Autodesk Fusion 360 part; units mm, degrees
(part 11 of 18)
sketch "Sketch1 (2)" plane through (0, 0, 0) normal (0, 0, 1) x (1, 0, 0) in component "Component"
  spline S0 degree 5 poles (24.241, -1.3145) (24.2412, -1.3145) (24.2415, -1.3145) (24.242, -1.3146) (24.2429, -1.3146) (24.2442, -1.3146) (24.2456, -1.3147) (24.2473, -1.3147) (24.2491, -1.3148) (24.2512, -1.3148) (24.2534, -1.3149) (24.2558, -1.3149) (24.2584, -1.315) (24.2611, -1.315) (24.2641, -1.3151) (24.2672, -1.3151) (24.2704, -1.3151) (24.2739, -1.3151) (24.2775, -1.3151) (24.2812, -1.3151) (24.2851, -1.3151) (24.2892, -1.315) (24.2934, -1.315) (24.2977, -1.3149) (24.3022, -1.3149) (24.3069, -1.3148) (24.3117, -1.3147) (24.3166, -1.3145) (24.3216, -1.3144) (24.3268, -1.3143) (24.3322, -1.3141) (24.3376, -1.3139) (24.3432, -1.3137) (24.3489, -1.3135) (24.3548, -1.3132) (24.3608, -1.313) (24.3669, -1.3127) (24.3731, -1.3124) (24.3794, -1.312) (24.3859, -1.3117) (24.3924, -1.3113) (24.3991, -1.3109) (24.4059, -1.3105) (24.4129, -1.3101) (24.4199, -1.3096) (24.427, -1.3091) (24.4343, -1.3086) (24.4416, -1.308) (24.4491, -1.3075) (24.4567, -1.3069) (24.4644, -1.3062) (24.4721, -1.3056) (24.48, -1.3049) (24.488, -1.3042) (24.4961, -1.3035) (24.5043, -1.3027) (24.5126, -1.3019) (24.521, -1.3011) (24.5294, -1.3003) (24.538, -1.2994) (24.5467, -1.2985) (24.5554, -1.2976) (24.5643, -1.2966) (24.5732, -1.2956) (24.5823, -1.2946) (24.5914, -1.2935) (24.6006, -1.2925) (24.6099, -1.2913) (24.6193, -1.2902) (24.6288, -1.289) (24.6383, -1.2878) (24.648, -1.2865) (24.6577, -1.2853) (24.6675, -1.284) (24.6774, -1.2826) (24.6874, -1.2812) (24.6974, -1.2798) (24.7076, -1.2784) (24.7178, -1.2769) (24.7281, -1.2754) (24.7385, -1.2738) (24.7489, -1.2723) (24.7594, -1.2707) (24.77, -1.269) (24.7807, -1.2673) (24.7915, -1.2656) (24.8023, -1.2638) (24.8132, -1.2621) (24.8242, -1.2602) (24.8352, -1.2584) (24.8464, -1.2565) (24.8575, -1.2545) (24.8688, -1.2526) (24.8801, -1.2506) (24.8915, -1.2485) (24.903, -1.2464) (24.9146, -1.2443) (24.9262, -1.2422) (24.9378, -1.24) (24.9496, -1.2378) (24.9614, -1.2355) (24.9733, -1.2332) (24.9852, -1.2308) (24.9972, -1.2285) (25.0093, -1.226) (25.0214, -1.2236) (25.0336, -1.2211) (25.0458, -1.2186) (25.0581, -1.216) (25.0705, -1.2134) (25.083, -1.2107) (25.0955, -1.2081) (25.108, -1.2053) (25.1206, -1.2026) (25.1333, -1.1998) (25.1461, -1.1969) (25.1589, -1.194) (25.1717, -1.1911) (25.1846, -1.1882) (25.1976, -1.1852) (25.2106, -1.1821) (25.2237, -1.179) (25.2368, -1.1759) (25.25, -1.1728) (25.2633, -1.1696) (25.2766, -1.1663) (25.2899, -1.163) (25.3034, -1.1597) (25.3168, -1.1564) (25.3303, -1.153) (25.3439, -1.1495) (25.3575, -1.146) (25.3712, -1.1425) (25.3849, -1.1389) (25.3987, -1.1353) (25.4125, -1.1317) (25.4264, -1.128) (25.4403, -1.1243) (25.4543, -1.1205) (25.4683, -1.1167) (25.4824, -1.1128) (25.4965, -1.1089) (25.5107, -1.105) (25.5249, -1.101) (25.5392, -1.097) (25.5535, -1.0929) (25.5679, -1.0888) (25.5823, -1.0846) (25.5967, -1.0805) (25.6112, -1.0762) (25.6258, -1.0719) (25.6404, -1.0676) (25.655, -1.0633) (25.6697, -1.0589) (25.6844, -1.0544) (25.6992, -1.0499) (25.714, -1.0454) (25.7288, -1.0408) (25.7437, -1.0362) (25.7587, -1.0316) (25.7736, -1.0268) (25.7887, -1.0221) (25.8037, -1.0173) (25.8188, -1.0125) (25.834, -1.0076) (25.8492, -1.0027) (25.8644, -0.9977) (25.8797, -0.9927) (25.895, -0.9877) (25.9103, -0.9826) (25.9257, -0.9775) (25.9411, -0.9723) (25.9566, -0.9671) (25.9721, -0.9618) (25.9876, -0.9565) (26.0032, -0.9511) (26.0188, -0.9457) (26.0345, -0.9403) (26.0502, -0.9348) (26.0659, -0.9293) (26.0817, -0.9237) (26.0975, -0.9181) (26.1133, -0.9124) (26.1292, -0.9067) (26.1451, -0.901) (26.161, -0.8952) (26.177, -0.8894) (26.193, -0.8835) (26.2091, -0.8776) (26.2252, -0.8716) (26.2413, -0.8656) (26.2574, -0.8595) (26.2736, -0.8534) (26.2898, -0.8473) (26.3061, -0.8411) (26.3224, -0.8349) (26.3387, -0.8286) (26.355, -0.8223) (26.3714, -0.8159) (26.3878, -0.8095) (26.4043, -0.803) (26.4207, -0.7965) (26.4373, -0.79) (26.4538, -0.7834) (26.4704, -0.7768) (26.487, -0.7701) (26.5036, -0.7633) (26.5202, -0.7566) (26.5369, -0.7498) (26.5537, -0.7429) (26.5704, -0.736) (26.5872, -0.7291) (26.604, -0.7221) (26.6208, -0.715) (26.6377, -0.7079) (26.6546, -0.7008) (26.6715, -0.6936) (26.6884, -0.6864) (26.7054, -0.6792) (26.7224, -0.6718) (26.7394, -0.6645) (26.7565, -0.6571) (26.7736, -0.6496) (26.7907, -0.6422) (26.8078, -0.6346) (26.825, -0.627) (26.8422, -0.6194) (26.8594, -0.6117) (26.8766, -0.604) (26.8939, -0.5963) (26.9112, -0.5885) (26.9285, -0.5806) (26.9458, -0.5727) (26.9632, -0.5648) (26.9806, -0.5568) (26.998, -0.5488) (27.0154, -0.5407) (27.0329, -0.5325) (27.0504, -0.5244) (27.0679, -0.5162) (27.0854, -0.5079) (27.0995, -0.5013) (27.11, -0.4963) (27.117, -0.4929) (27.1206, -0.4912) knots 0 0 0 0 0 0 0.00416667 0.00833333 0.0125 0.01666667 0.02083333 0.025 0.02916667 0.03333333 0.0375 0.04166667 0.04583333 0.05 0.05416667 0.05833333 0.0625 0.06666667 0.07083333 0.075 0.07916667 0.08333333 0.0875 0.09166667 0.09583333 0.1 0.10416667 0.10833333 0.1125 0.11666667 0.12083333 0.125 0.12916667 0.13333333 0.1375 0.14166667 0.14583333 0.15 0.15416667 0.15833333 0.1625 0.16666667 0.17083333 0.175 0.17916667 0.18333333 0.1875 0.19166667 0.19583333 0.2 0.20416667 0.20833333 0.2125 0.21666667 0.22083333 0.225 0.22916667 0.23333333 0.2375 0.24166667 0.24583333 0.25 0.25416667 0.25833333 0.2625 0.26666667 0.27083333 0.275 0.27916667 0.28333333 0.2875 0.29166667 0.29583333 0.3 0.30416667 0.30833333 0.3125 0.31666667 0.32083333 0.325 0.32916667 0.33333333 0.3375 0.34166667 0.34583333 0.35 0.35416667 0.35833333 0.3625 0.36666667 0.37083333 0.375 0.37916667 0.38333333 0.3875 0.39166667 0.39583333 0.4 0.40416667 0.40833333 0.4125 0.41666667 0.42083333 0.425 0.42916667 0.43333333 0.4375 0.44166667 0.44583333 0.45 0.45416667 0.45833333 0.4625 0.46666667 0.47083333 0.475 0.47916667 0.48333333 0.4875 0.49166667 0.49583333 0.5 0.50416667 0.50833333 0.5125 0.51666667 0.52083333 0.525 0.52916667 0.53333333 0.5375 0.54166667 0.54583333 0.55 0.55416667 0.55833333 0.5625 0.56666667 0.57083333 0.575 0.57916667 0.58333333 0.5875 0.59166667 0.59583333 0.6 0.60416667 0.60833333 0.6125 0.61666667 0.62083333 0.625 0.62916667 0.63333333 0.6375 0.64166667 0.64583333 0.65 0.65416667 0.65833333 0.6625 0.66666667 0.67083333 0.675 0.67916667 0.68333333 0.6875 0.69166667 0.69583333 0.7 0.70416667 0.70833333 0.7125 0.71666667 0.72083333 0.725 0.72916667 0.73333333 0.7375 0.74166667 0.74583333 0.75 0.75416667 0.75833333 0.7625 0.76666667 0.77083333 0.775 0.77916667 0.78333333 0.7875 0.79166667 0.79583333 0.8 0.80416667 0.80833333 0.8125 0.81666667 0.82083333 0.825 0.82916667 0.83333333 0.8375 0.84166667 0.84583333 0.85 0.85416667 0.85833333 0.8625 0.86666667 0.87083333 0.875 0.87916667 0.88333333 0.8875 0.89166667 0.89583333 0.9 0.90416667 0.90833333 0.9125 0.91666667 0.92083333 0.925 0.92916667 0.93333333 0.9375 0.94166667 0.94583333 0.95 0.95416667 0.95833333 0.9625 0.96666667 0.97083333 0.975 0.97916667 0.98333333 0.9875 0.99166667 0.99583333 1 1 1 1 1 1
  spline S1 degree 5 poles (24.241, 1.3145) (24.2412, 1.3145) (24.2415, 1.3145) (24.242, 1.3146) (24.2429, 1.3146) (24.2442, 1.3146) (24.2456, 1.3147) (24.2473, 1.3147) (24.2491, 1.3148) (24.2512, 1.3148) (24.2534, 1.3149) (24.2558, 1.3149) (24.2584, 1.315) (24.2611, 1.315) (24.2641, 1.3151) (24.2672, 1.3151) (24.2704, 1.3151) (24.2739, 1.3151) (24.2775, 1.3151) (24.2812, 1.3151) (24.2851, 1.3151) (24.2892, 1.315) (24.2934, 1.315) (24.2977, 1.3149) (24.3022, 1.3149) (24.3069, 1.3148) (24.3117, 1.3147) (24.3166, 1.3145) (24.3216, 1.3144) (24.3268, 1.3143) (24.3322, 1.3141) (24.3376, 1.3139) (24.3432, 1.3137) (24.3489, 1.3135) (24.3548, 1.3132) (24.3608, 1.313) (24.3669, 1.3127) (24.3731, 1.3124) (24.3794, 1.312) (24.3859, 1.3117) (24.3924, 1.3113) (24.3991, 1.3109) (24.4059, 1.3105) (24.4129, 1.3101) (24.4199, 1.3096) (24.427, 1.3091) (24.4343, 1.3086) (24.4416, 1.308) (24.4491, 1.3075) (24.4567, 1.3069) (24.4644, 1.3062) (24.4721, 1.3056) (24.48, 1.3049) (24.488, 1.3042) (24.4961, 1.3035) (24.5043, 1.3027) (24.5126, 1.3019) (24.521, 1.3011) (24.5294, 1.3003) (24.538, 1.2994) (24.5467, 1.2985) (24.5554, 1.2976) (24.5643, 1.2966) (24.5732, 1.2956) (24.5823, 1.2946) (24.5914, 1.2935) (24.6006, 1.2925) (24.6099, 1.2913) (24.6193, 1.2902) (24.6288, 1.289) (24.6383, 1.2878) (24.648, 1.2865) (24.6577, 1.2853) (24.6675, 1.284) (24.6774, 1.2826) (24.6874, 1.2812) (24.6974, 1.2798) (24.7076, 1.2784) (24.7178, 1.2769) (24.7281, 1.2754) (24.7385, 1.2738) (24.7489, 1.2723) (24.7594, 1.2707) (24.77, 1.269) (24.7807, 1.2673) (24.7915, 1.2656) (24.8023, 1.2638) (24.8132, 1.2621) (24.8242, 1.2602) (24.8352, 1.2584) (24.8464, 1.2565) (24.8575, 1.2545) (24.8688, 1.2526) (24.8801, 1.2506) (24.8915, 1.2485) (24.903, 1.2464) (24.9146, 1.2443) (24.9262, 1.2422) (24.9378, 1.24) (24.9496, 1.2378) (24.9614, 1.2355) (24.9733, 1.2332) (24.9852, 1.2308) (24.9972, 1.2285) (25.0093, 1.226) (25.0214, 1.2236) (25.0336, 1.2211) (25.0458, 1.2186) (25.0581, 1.216) (25.0705, 1.2134) (25.083, 1.2107) (25.0955, 1.2081) (25.108, 1.2053) (25.1206, 1.2026) (25.1333, 1.1998) (25.1461, 1.1969) (25.1589, 1.194) (25.1717, 1.1911) (25.1846, 1.1882) (25.1976, 1.1852) (25.2106, 1.1821) (25.2237, 1.179) (25.2368, 1.1759) (25.25, 1.1728) (25.2633, 1.1696) (25.2766, 1.1663) (25.2899, 1.163) (25.3034, 1.1597) (25.3168, 1.1564) (25.3303, 1.153) (25.3439, 1.1495) (25.3575, 1.146) (25.3712, 1.1425) (25.3849, 1.1389) (25.3987, 1.1353) (25.4125, 1.1317) (25.4264, 1.128) (25.4403, 1.1243) (25.4543, 1.1205) (25.4683, 1.1167) (25.4824, 1.1128) (25.4965, 1.1089) (25.5107, 1.105) (25.5249, 1.101) (25.5392, 1.097) (25.5535, 1.0929) (25.5679, 1.0888) (25.5823, 1.0846) (25.5967, 1.0805) (25.6112, 1.0762) (25.6258, 1.0719) (25.6404, 1.0676) (25.655, 1.0633) (25.6697, 1.0589) (25.6844, 1.0544) (25.6992, 1.0499) (25.714, 1.0454) (25.7288, 1.0408) (25.7437, 1.0362) (25.7587, 1.0316) (25.7736, 1.0268) (25.7887, 1.0221) (25.8037, 1.0173) (25.8188, 1.0125) (25.834, 1.0076) (25.8492, 1.0027) (25.8644, 0.9977) (25.8797, 0.9927) (25.895, 0.9877) (25.9103, 0.9826) (25.9257, 0.9775) (25.9411, 0.9723) (25.9566, 0.9671) (25.9721, 0.9618) (25.9876, 0.9565) (26.0032, 0.9511) (26.0188, 0.9457) (26.0345, 0.9403) (26.0502, 0.9348) (26.0659, 0.9293) (26.0817, 0.9237) (26.0975, 0.9181) (26.1133, 0.9124) (26.1292, 0.9067) (26.1451, 0.901) (26.161, 0.8952) (26.177, 0.8894) (26.193, 0.8835) (26.2091, 0.8776) (26.2252, 0.8716) (26.2413, 0.8656) (26.2574, 0.8595) (26.2736, 0.8534) (26.2898, 0.8473) (26.3061, 0.8411) (26.3224, 0.8349) (26.3387, 0.8286) (26.355, 0.8223) (26.3714, 0.8159) (26.3878, 0.8095) (26.4043, 0.803) (26.4207, 0.7965) (26.4373, 0.79) (26.4538, 0.7834) (26.4704, 0.7768) (26.487, 0.7701) (26.5036, 0.7633) (26.5202, 0.7566) (26.5369, 0.7498) (26.5537, 0.7429) (26.5704, 0.736) (26.5872, 0.7291) (26.604, 0.7221) (26.6208, 0.715) (26.6377, 0.7079) (26.6546, 0.7008) (26.6715, 0.6936) (26.6884, 0.6864) (26.7054, 0.6792) (26.7224, 0.6718) (26.7394, 0.6645) (26.7565, 0.6571) (26.7736, 0.6496) (26.7907, 0.6422) (26.8078, 0.6346) (26.825, 0.627) (26.8422, 0.6194) (26.8594, 0.6117) (26.8766, 0.604) (26.8939, 0.5963) (26.9112, 0.5885) (26.9285, 0.5806) (26.9458, 0.5727) (26.9632, 0.5648) (26.9806, 0.5568) (26.998, 0.5488) (27.0154, 0.5407) (27.0329, 0.5325) (27.0504, 0.5244) (27.0679, 0.5162) (27.0854, 0.5079) (27.0995, 0.5013) (27.11, 0.4963) (27.117, 0.4929) (27.1206, 0.4912) knots 0 0 0 0 0 0 0.00416667 0.00833333 0.0125 0.01666667 0.02083333 0.025 0.02916667 0.03333333 0.0375 0.04166667 0.04583333 0.05 0.05416667 0.05833333 0.0625 0.06666667 0.07083333 0.075 0.07916667 0.08333333 0.0875 0.09166667 0.09583333 0.1 0.10416667 0.10833333 0.1125 0.11666667 0.12083333 0.125 0.12916667 0.13333333 0.1375 0.14166667 0.14583333 0.15 0.15416667 0.15833333 0.1625 0.16666667 0.17083333 0.175 0.17916667 0.18333333 0.1875 0.19166667 0.19583333 0.2 0.20416667 0.20833333 0.2125 0.21666667 0.22083333 0.225 0.22916667 0.23333333 0.2375 0.24166667 0.24583333 0.25 0.25416667 0.25833333 0.2625 0.26666667 0.27083333 0.275 0.27916667 0.28333333 0.2875 0.29166667 0.29583333 0.3 0.30416667 0.30833333 0.3125 0.31666667 0.32083333 0.325 0.32916667 0.33333333 0.3375 0.34166667 0.34583333 0.35 0.35416667 0.35833333 0.3625 0.36666667 0.37083333 0.375 0.37916667 0.38333333 0.3875 0.39166667 0.39583333 0.4 0.40416667 0.40833333 0.4125 0.41666667 0.42083333 0.425 0.42916667 0.43333333 0.4375 0.44166667 0.44583333 0.45 0.45416667 0.45833333 0.4625 0.46666667 0.47083333 0.475 0.47916667 0.48333333 0.4875 0.49166667 0.49583333 0.5 0.50416667 0.50833333 0.5125 0.51666667 0.52083333 0.525 0.52916667 0.53333333 0.5375 0.54166667 0.54583333 0.55 0.55416667 0.55833333 0.5625 0.56666667 0.57083333 0.575 0.57916667 0.58333333 0.5875 0.59166667 0.59583333 0.6 0.60416667 0.60833333 0.6125 0.61666667 0.62083333 0.625 0.62916667 0.63333333 0.6375 0.64166667 0.64583333 0.65 0.65416667 0.65833333 0.6625 0.66666667 0.67083333 0.675 0.67916667 0.68333333 0.6875 0.69166667 0.69583333 0.7 0.70416667 0.70833333 0.7125 0.71666667 0.72083333 0.725 0.72916667 0.73333333 0.7375 0.74166667 0.74583333 0.75 0.75416667 0.75833333 0.7625 0.76666667 0.77083333 0.775 0.77916667 0.78333333 0.7875 0.79166667 0.79583333 0.8 0.80416667 0.80833333 0.8125 0.81666667 0.82083333 0.825 0.82916667 0.83333333 0.8375 0.84166667 0.84583333 0.85 0.85416667 0.85833333 0.8625 0.86666667 0.87083333 0.875 0.87916667 0.88333333 0.8875 0.89166667 0.89583333 0.9 0.90416667 0.90833333 0.9125 0.91666667 0.92083333 0.925 0.92916667 0.93333333 0.9375 0.94166667 0.94583333 0.95 0.95416667 0.95833333 0.9625 0.96666667 0.97083333 0.975 0.97916667 0.98333333 0.9875 0.99166667 0.99583333 1 1 1 1 1 1
  spline S2 degree 5 poles (24.2398, -1.3145) (24.2398, -1.3145) (24.2399, -1.3145) (24.2401, -1.3145) (24.2403, -1.3145) (24.2405, -1.3145) (24.2407, -1.3145) (24.2409, -1.3145) (24.241, -1.3145) (24.241, -1.3145) knots 0 0 0 0 0 0 0.2 0.4 0.6 0.8 1 1 1 1 1 1
  spline S3 degree 5 poles (24.2398, 1.3145) (24.2398, 1.3145) (24.2399, 1.3145) (24.2401, 1.3145) (24.2403, 1.3145) (24.2405, 1.3145) (24.2407, 1.3145) (24.2409, 1.3145) (24.241, 1.3145) (24.241, 1.3145) knots 0 0 0 0 0 0 0.2 0.4 0.6 0.8 1 1 1 1 1 1
  line L0 (0, 0) -> (24.2398, -1.3145)
  line L1 (0, 0) -> (24.2398, 1.3145)
  arc A0 (27.1206, -0.4912) -> (27.1206, 0.4912) centre (0, 0) ccw
  point P0 (24.2448, -1.3147)
  point P1 (24.2511, -1.3148)
  point P2 (24.2599, -1.315)
  point P3 (24.2712, -1.3151)
  point P4 (24.285, -1.3151)
  point P5 (24.3013, -1.3149)
  point P6 (24.3202, -1.3145)
  point P7 (24.3415, -1.3138)
  point P8 (24.3654, -1.3127)
  point P9 (24.3917, -1.3114)
  point P10 (24.4206, -1.3095)
  point P11 (24.4519, -1.3072)
  point P12 (24.4857, -1.3044)
  point P13 (24.522, -1.301)
  point P14 (24.5607, -1.297)
  point P15 (24.6019, -1.2923)
  point P16 (24.6456, -1.2869)
  point P17 (24.6916, -1.2806)
  point P18 (24.7401, -1.2736)
  point P19 (24.791, -1.2657)
  point P20 (24.8443, -1.2568)
  point P21 (24.9, -1.247)
  point P22 (24.9581, -1.2361)
  point P23 (25.0185, -1.2242)
  point P24 (25.0812, -1.2111)
  point P25 (25.1463, -1.1969)
  point P26 (25.2136, -1.1814)
  point P27 (25.2832, -1.1647)
  point P28 (25.3552, -1.1466)
  point P29 (25.4293, -1.1272)
  point P30 (25.5057, -1.1064)
  point P31 (25.5842, -1.0841)
  point P32 (25.665, -1.0603)
  point P33 (25.7479, -1.0349)
  point P34 (25.8329, -1.0079)
  point P35 (25.9201, -0.9793)
  point P36 (26.0093, -0.949)
  point P37 (26.1006, -0.917)
  point P38 (26.1939, -0.8832)
  point P39 (26.2892, -0.8475)
  point P40 (26.3865, -0.81)
  point P41 (26.4858, -0.7705)
  point P42 (26.587, -0.7291)
  point P43 (26.69, -0.6857)
  point P44 (26.795, -0.6403)
  point P45 (26.9017, -0.5927)
  point P46 (27.0102, -0.5431)
  point P47 (24.2448, 1.3147)
  point P48 (24.2511, 1.3148)
  point P49 (24.2599, 1.315)
  point P50 (24.2712, 1.3151)
  point P51 (24.285, 1.3151)
  point P52 (24.3013, 1.3149)
  point P53 (24.3202, 1.3145)
  point P54 (24.3415, 1.3138)
  point P55 (24.3654, 1.3127)
  point P56 (24.3917, 1.3114)
  point P57 (24.4206, 1.3095)
  point P58 (24.4519, 1.3072)
  point P59 (24.4857, 1.3044)
  point P60 (24.522, 1.301)
  point P61 (24.5607, 1.297)
  point P62 (24.6019, 1.2923)
  point P63 (24.6456, 1.2869)
  point P64 (24.6916, 1.2806)
  point P65 (24.7401, 1.2736)
  point P66 (24.791, 1.2657)
  point P67 (24.8443, 1.2568)
  point P68 (24.9, 1.247)
  point P69 (24.9581, 1.2361)
  point P70 (25.0185, 1.2242)
  point P71 (25.0812, 1.2111)
  point P72 (25.1463, 1.1969)
  point P73 (25.2136, 1.1814)
  point P74 (25.2832, 1.1647)
  point P75 (25.3552, 1.1466)
  point P76 (25.4293, 1.1272)
  point P77 (25.5057, 1.1064)
  point P78 (25.5842, 1.0841)
  point P79 (25.665, 1.0603)
  point P80 (25.7479, 1.0349)
  point P81 (25.8329, 1.0079)
  point P82 (25.9201, 0.9793)
  point P83 (26.0093, 0.949)
  point P84 (26.1006, 0.917)
  point P85 (26.1939, 0.8832)
  point P86 (26.2892, 0.8475)
  point P87 (26.3865, 0.81)
  point P88 (26.4858, 0.7705)
  point P89 (26.587, 0.7291)
  point P90 (26.69, 0.6857)
  point P91 (26.795, 0.6403)
  point P92 (26.9017, 0.5927)
  point P93 (27.0102, 0.5431)
sketch "Sketch2" plane through (0, 0, 0) normal (0, 0, 1) x (1, 0, 0) in component "Component"
  circle A0 centre (0, 0) radius 24.2188
extrude "Extrude1" add sketch "Sketch2" along normal blind 3 makes body 1 in component "Component"
extrude "Extrude2" add sketch "Sketch1 (2)" along normal blind 3 separate body makes body 2 in component "Component"
pattern_circular "C-Pattern1" count 40 over 360 about axis through (0, 0, 1.75) along (0, 0, 1) of "Extrude2" makes body 3 at (8.0494, 0.8313, 1) makes body 4 at (7.5495, 2.9137, 1) makes body 5 at (7.0007, 4.0588, 1) makes body 6 at (6.7947, 4.395, 1) makes body 7 at (6.0235, 5.4038, 1) makes body 8 at (5.104, 6.2796, 1) makes body 9 at (3.278, 7.3986, 1) makes body 10 at (2.9137, 7.5495, 2) makes body 11 at (0.8313, 8.0494, 1) makes body 12 at (0.4382, 8.0803, 1) makes body 13 at (-0.8313, 8.0494, 1) makes body 14 at (-2.9137, 7.5495, 1) makes body 15 at (-3.278, 7.3986, 1) makes body 16 at (-4.395, 6.7947, 1) makes body 17 at (-5.4038, 6.0235, 1) makes body 18 at (-6.2796, 5.104, 1) makes body 19 at (-7.3986, 3.278, 1) makes body 20 at (-7.8203, 2.0802, 1) makes body 21 at (-8.0494, 0.8313, 1) makes body 22 at (-8.0803, 0.4382, 1) makes body 23 at (-8.0494, -0.8313, 1) makes body 24 at (-7.8203, -2.0802, 1) makes body 25 at (-7.3986, -3.278, 1) makes body 26 at (-6.7947, -4.395, 1) makes body 27 at (-6.0235, -5.4038, 1) makes body 28 at (-4.395, -6.7947, 1) makes body 29 at (-4.0588, -7.0007, 1) makes body 30 at (-2.9137, -7.5495, 2) makes body 31 at (-0.8313, -8.0494, 1) makes body 32 at (-0.4382, -8.0803, 1) makes body 33 at (0.8313, -8.0494, 1) makes body 34 at (2.0802, -7.8203, 1) makes body 35 at (3.278, -7.3986, 1) makes body 36 at (4.395, -6.7947, 1) makes body 37 at (5.4038, -6.0235, 1) makes body 38 at (6.2796, -5.104, 1) makes body 39 at (7.0007, -4.0588, 1) makes body 40 at (7.8203, -2.0802, 1) makes body 41 at (8.0494, -0.8313, 1) in component "Component"
combine "Combine1" operation add target body 1 tool bodies 2 3 4 5 6 7 8 9 10 11 12 13 14 15 16 17 18 19 20 21 22 23 24 25 26 27 28 29 30 31 32 33 34 35 36 37 38 39 40 41 in component "Component"
sketch "Sketch3" plane through (0, 0, 0) normal (0, 0, 1) x (1, 0, 0) in component "Component"
  line L0 (0, 0) -> (52.4707, 0) construction
  line L1 (52.4707, 0) -> (52.4707, 3) construction
  line L2 (52.4707, 3) -> (0, 3) construction
  line L3 (0, 3) -> (0, 0) construction
  constraint perpendicular L0 L1
  constraint parallel L0 L2
  constraint parallel L1 L3
extrude "Extrude3" cut sketch "Sketch1" against normal blind 6 contours L120 L121 A62 | L120 L122 A62 | L121 L122 A62 | A61 | A63 | A64 | A65 | A66 | A67 | A68 | A69 | A70 | A71 | A72 bodies 1 in component "Component"
component "Component" placed x (1, 0, 0) y (0, 1, 0) z (0, 0, 1) at (0, 0, 0)

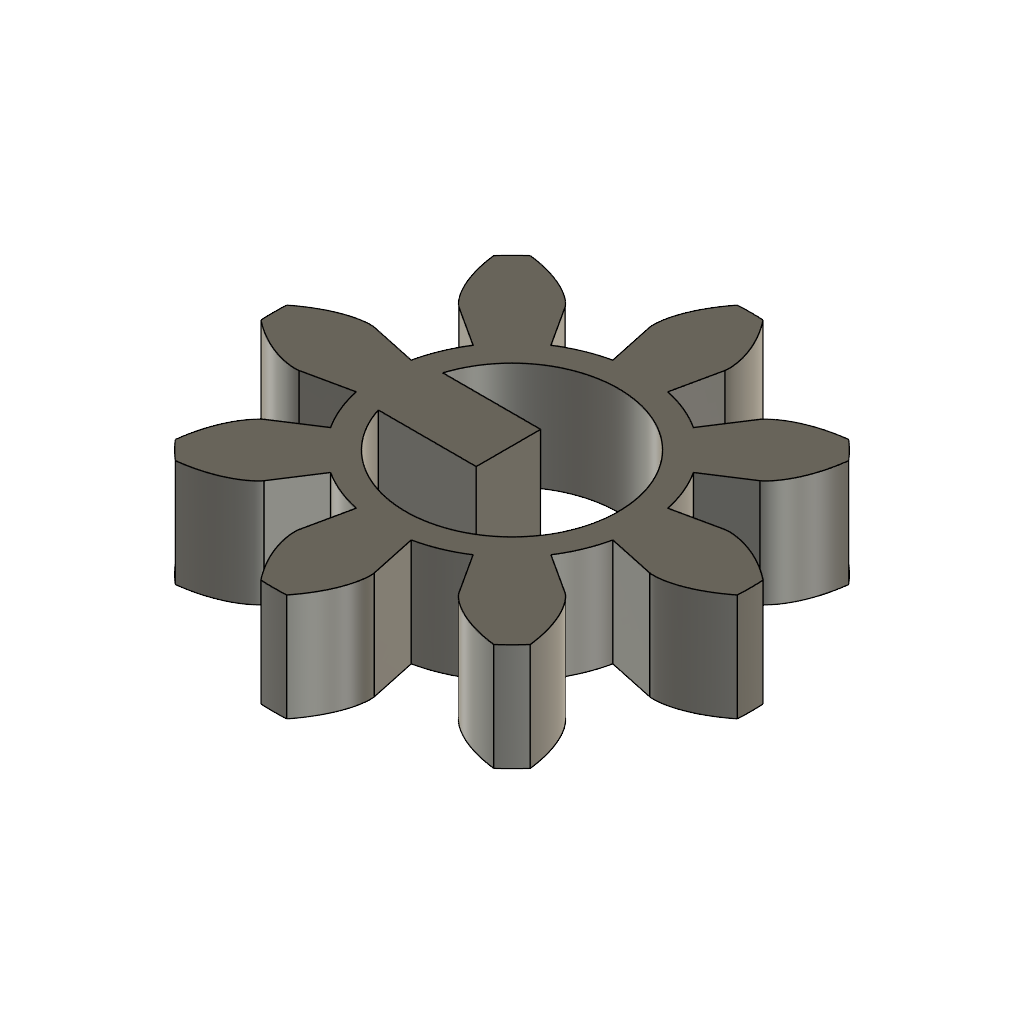
design "dispenser-driven-gear"
part number: 2026-07-25-20-51-35-213
part number: 2026-09-10-19-47-47-084
Autodesk Fusion 360 part; units mm, degrees
sketch "Sketch1" plane through (0, 0, 0) normal (0, 0, 1) x (1, 0, 0) in component "Component"
  spline S0 degree 5 poles (4.9011, -1.051) (4.9011, -1.0511) (4.9013, -1.0511) (4.9016, -1.0512) (4.9021, -1.0512) (4.9028, -1.0514) (4.9036, -1.0515) (4.9045, -1.0517) (4.9055, -1.0518) (4.9066, -1.052) (4.9078, -1.0522) (4.9092, -1.0524) (4.9106, -1.0526) (4.9121, -1.0529) (4.9137, -1.0531) (4.9154, -1.0533) (4.9172, -1.0536) (4.9191, -1.0538) (4.9211, -1.054) (4.9232, -1.0543) (4.9254, -1.0545) (4.9277, -1.0548) (4.9301, -1.055) (4.9325, -1.0553) (4.9351, -1.0555) (4.9377, -1.0558) (4.9404, -1.056) (4.9432, -1.0562) (4.9461, -1.0564) (4.9491, -1.0567) (4.9521, -1.0569) (4.9553, -1.0571) (4.9585, -1.0573) (4.9618, -1.0575) (4.9652, -1.0576) (4.9687, -1.0578) (4.9722, -1.058) (4.9758, -1.0581) (4.9795, -1.0582) (4.9833, -1.0583) (4.9872, -1.0584) (4.9911, -1.0585) (4.9951, -1.0586) (4.9992, -1.0587) (5.0033, -1.0587) (5.0075, -1.0587) (5.0118, -1.0587) (5.0162, -1.0587) (5.0206, -1.0587) (5.0251, -1.0587) (5.0297, -1.0586) (5.0344, -1.0585) (5.0391, -1.0584) (5.0439, -1.0583) (5.0487, -1.0581) (5.0536, -1.058) (5.0586, -1.0578) (5.0637, -1.0576) (5.0688, -1.0573) (5.074, -1.0571) (5.0792, -1.0568) (5.0845, -1.0565) (5.0899, -1.0561) (5.0953, -1.0558) (5.1008, -1.0554) (5.1063, -1.055) (5.112, -1.0545) (5.1176, -1.0541) (5.1234, -1.0536) (5.1291, -1.0531) (5.135, -1.0525) (5.1409, -1.0519) (5.1469, -1.0513) (5.1529, -1.0507) (5.159, -1.05) (5.1651, -1.0493) (5.1713, -1.0486) (5.1775, -1.0479) (5.1838, -1.0471) (5.1902, -1.0463) (5.1966, -1.0454) (5.203, -1.0446) (5.2095, -1.0436) (5.2161, -1.0427) (5.2227, -1.0417) (5.2294, -1.0407) (5.2361, -1.0397) (5.2428, -1.0386) (5.2496, -1.0375) (5.2565, -1.0364) (5.2634, -1.0352) (5.2704, -1.034) (5.2774, -1.0327) (5.2844, -1.0314) (5.2915, -1.0301) (5.2987, -1.0288) (5.3059, -1.0274) (5.3131, -1.026) (5.3204, -1.0245) (5.3277, -1.023) (5.3351, -1.0215) (5.3425, -1.0199) (5.3499, -1.0183) (5.3574, -1.0167) (5.365, -1.015) (5.3726, -1.0133) (5.3802, -1.0115) (5.3879, -1.0097) (5.3956, -1.0079) (5.4033, -1.006) (5.4111, -1.0041) (5.4189, -1.0021) (5.4268, -1.0001) (5.4347, -0.9981) (5.4427, -0.996) (5.4506, -0.9939) (5.4587, -0.9918) (5.4667, -0.9896) (5.4748, -0.9874) (5.483, -0.9851) (5.4911, -0.9828) (5.4993, -0.9804) (5.5076, -0.978) (5.5159, -0.9756) (5.5242, -0.9731) (5.5325, -0.9706) (5.5409, -0.968) (5.5493, -0.9654) (5.5577, -0.9628) (5.5662, -0.9601) (5.5747, -0.9574) (5.5833, -0.9546) (5.5919, -0.9518) (5.6005, -0.9489) (5.6091, -0.946) (5.6178, -0.9431) (5.6265, -0.9401) (5.6352, -0.9371) (5.644, -0.934) (5.6528, -0.9309) (5.6616, -0.9277) (5.6704, -0.9245) (5.6793, -0.9213) (5.6882, -0.918) (5.6971, -0.9146) (5.7061, -0.9113) (5.7151, -0.9078) (5.7241, -0.9044) (5.7331, -0.9008) (5.7422, -0.8973) (5.7513, -0.8937) (5.7604, -0.89) (5.7695, -0.8863) (5.7787, -0.8826) (5.7879, -0.8788) (5.7971, -0.875) (5.8063, -0.8711) (5.8156, -0.8672) (5.8249, -0.8632) (5.8342, -0.8592) (5.8435, -0.8551) (5.8529, -0.851) (5.8622, -0.8469) (5.8716, -0.8427) (5.881, -0.8384) (5.8905, -0.8341) (5.8999, -0.8298) (5.9094, -0.8254) (5.9189, -0.821) (5.9284, -0.8165) (5.938, -0.812) (5.9475, -0.8074) (5.9571, -0.8028) (5.9667, -0.7981) (5.9763, -0.7934) (5.9859, -0.7887) (5.9956, -0.7839) (6.0052, -0.779) (6.0149, -0.7741) (6.0246, -0.7692) (6.0343, -0.7642) (6.044, -0.7591) (6.0538, -0.754) (6.0635, -0.7489) (6.0733, -0.7437) (6.0831, -0.7385) (6.0929, -0.7332) (6.1027, -0.7279) (6.1126, -0.7225) (6.1224, -0.7171) (6.1323, -0.7116) (6.1421, -0.7061) (6.152, -0.7005) (6.1619, -0.6949) (6.1718, -0.6893) (6.1818, -0.6836) (6.1917, -0.6778) (6.2016, -0.672) (6.2116, -0.6661) (6.2216, -0.6602) (6.2316, -0.6543) (6.2415, -0.6483) (6.2515, -0.6423) (6.2616, -0.6362) (6.2716, -0.63) (6.2816, -0.6238) (6.2916, -0.6176) (6.3017, -0.6113) (6.3117, -0.605) (6.3218, -0.5986) (6.3319, -0.5921) (6.342, -0.5857) (6.3521, -0.5791) (6.3621, -0.5726) (6.3722, -0.5659) (6.3824, -0.5593) (6.3925, -0.5525) (6.4026, -0.5458) (6.4127, -0.5389) (6.4229, -0.5321) (6.433, -0.5252) (6.4431, -0.5182) (6.4533, -0.5112) (6.4634, -0.5041) (6.4736, -0.497) (6.4838, -0.4898) (6.4939, -0.4826) (6.5041, -0.4754) (6.5143, -0.4681) (6.5244, -0.4607) (6.5346, -0.4533) (6.5448, -0.4459) (6.555, -0.4384) (6.5652, -0.4308) (6.5754, -0.4232) (6.5855, -0.4156) (6.5957, -0.4079) (6.6059, -0.4001) (6.6161, -0.3923) (6.6263, -0.3845) (6.6365, -0.3766) (6.6447, -0.3702) (6.6508, -0.3655) (6.6549, -0.3623) (6.6569, -0.3607) knots 0 0 0 0 0 0 0.00416667 0.00833333 0.0125 0.01666667 0.02083333 0.025 0.02916667 0.03333333 0.0375 0.04166667 0.04583333 0.05 0.05416667 0.05833333 0.0625 0.06666667 0.07083333 0.075 0.07916667 0.08333333 0.0875 0.09166667 0.09583333 0.1 0.10416667 0.10833333 0.1125 0.11666667 0.12083333 0.125 0.12916667 0.13333333 0.1375 0.14166667 0.14583333 0.15 0.15416667 0.15833333 0.1625 0.16666667 0.17083333 0.175 0.17916667 0.18333333 0.1875 0.19166667 0.19583333 0.2 0.20416667 0.20833333 0.2125 0.21666667 0.22083333 0.225 0.22916667 0.23333333 0.2375 0.24166667 0.24583333 0.25 0.25416667 0.25833333 0.2625 0.26666667 0.27083333 0.275 0.27916667 0.28333333 0.2875 0.29166667 0.29583333 0.3 0.30416667 0.30833333 0.3125 0.31666667 0.32083333 0.325 0.32916667 0.33333333 0.3375 0.34166667 0.34583333 0.35 0.35416667 0.35833333 0.3625 0.36666667 0.37083333 0.375 0.37916667 0.38333333 0.3875 0.39166667 0.39583333 0.4 0.40416667 0.40833333 0.4125 0.41666667 0.42083333 0.425 0.42916667 0.43333333 0.4375 0.44166667 0.44583333 0.45 0.45416667 0.45833333 0.4625 0.46666667 0.47083333 0.475 0.47916667 0.48333333 0.4875 0.49166667 0.49583333 0.5 0.50416667 0.50833333 0.5125 0.51666667 0.52083333 0.525 0.52916667 0.53333333 0.5375 0.54166667 0.54583333 0.55 0.55416667 0.55833333 0.5625 0.56666667 0.57083333 0.575 0.57916667 0.58333333 0.5875 0.59166667 0.59583333 0.6 0.60416667 0.60833333 0.6125 0.61666667 0.62083333 0.625 0.62916667 0.63333333 0.6375 0.64166667 0.64583333 0.65 0.65416667 0.65833333 0.6625 0.66666667 0.67083333 0.675 0.67916667 0.68333333 0.6875 0.69166667 0.69583333 0.7 0.70416667 0.70833333 0.7125 0.71666667 0.72083333 0.725 0.72916667 0.73333333 0.7375 0.74166667 0.74583333 0.75 0.75416667 0.75833333 0.7625 0.76666667 0.77083333 0.775 0.77916667 0.78333333 0.7875 0.79166667 0.79583333 0.8 0.80416667 0.80833333 0.8125 0.81666667 0.82083333 0.825 0.82916667 0.83333333 0.8375 0.84166667 0.84583333 0.85 0.85416667 0.85833333 0.8625 0.86666667 0.87083333 0.875 0.87916667 0.88333333 0.8875 0.89166667 0.89583333 0.9 0.90416667 0.90833333 0.9125 0.91666667 0.92083333 0.925 0.92916667 0.93333333 0.9375 0.94166667 0.94583333 0.95 0.95416667 0.95833333 0.9625 0.96666667 0.97083333 0.975 0.97916667 0.98333333 0.9875 0.99166667 0.99583333 1 1 1 1 1 1
  spline S1 degree 5 poles (4.9011, 1.051) (4.9011, 1.0511) (4.9013, 1.0511) (4.9016, 1.0512) (4.9021, 1.0512) (4.9028, 1.0514) (4.9036, 1.0515) (4.9045, 1.0517) (4.9055, 1.0518) (4.9066, 1.052) (4.9078, 1.0522) (4.9092, 1.0524) (4.9106, 1.0526) (4.9121, 1.0529) (4.9137, 1.0531) (4.9154, 1.0533) (4.9172, 1.0536) (4.9191, 1.0538) (4.9211, 1.054) (4.9232, 1.0543) (4.9254, 1.0545) (4.9277, 1.0548) (4.9301, 1.055) (4.9325, 1.0553) (4.9351, 1.0555) (4.9377, 1.0558) (4.9404, 1.056) (4.9432, 1.0562) (4.9461, 1.0564) (4.9491, 1.0567) (4.9521, 1.0569) (4.9553, 1.0571) (4.9585, 1.0573) (4.9618, 1.0575) (4.9652, 1.0576) (4.9687, 1.0578) (4.9722, 1.058) (4.9758, 1.0581) (4.9795, 1.0582) (4.9833, 1.0583) (4.9872, 1.0584) (4.9911, 1.0585) (4.9951, 1.0586) (4.9992, 1.0587) (5.0033, 1.0587) (5.0075, 1.0587) (5.0118, 1.0587) (5.0162, 1.0587) (5.0206, 1.0587) (5.0251, 1.0587) (5.0297, 1.0586) (5.0344, 1.0585) (5.0391, 1.0584) (5.0439, 1.0583) (5.0487, 1.0581) (5.0536, 1.058) (5.0586, 1.0578) (5.0637, 1.0576) (5.0688, 1.0573) (5.074, 1.0571) (5.0792, 1.0568) (5.0845, 1.0565) (5.0899, 1.0561) (5.0953, 1.0558) (5.1008, 1.0554) (5.1063, 1.055) (5.112, 1.0545) (5.1176, 1.0541) (5.1234, 1.0536) (5.1291, 1.0531) (5.135, 1.0525) (5.1409, 1.0519) (5.1469, 1.0513) (5.1529, 1.0507) (5.159, 1.05) (5.1651, 1.0493) (5.1713, 1.0486) (5.1775, 1.0479) (5.1838, 1.0471) (5.1902, 1.0463) (5.1966, 1.0454) (5.203, 1.0446) (5.2095, 1.0436) (5.2161, 1.0427) (5.2227, 1.0417) (5.2294, 1.0407) (5.2361, 1.0397) (5.2428, 1.0386) (5.2496, 1.0375) (5.2565, 1.0364) (5.2634, 1.0352) (5.2704, 1.034) (5.2774, 1.0327) (5.2844, 1.0314) (5.2915, 1.0301) (5.2987, 1.0288) (5.3059, 1.0274) (5.3131, 1.026) (5.3204, 1.0245) (5.3277, 1.023) (5.3351, 1.0215) (5.3425, 1.0199) (5.3499, 1.0183) (5.3574, 1.0167) (5.365, 1.015) (5.3726, 1.0133) (5.3802, 1.0115) (5.3879, 1.0097) (5.3956, 1.0079) (5.4033, 1.006) (5.4111, 1.0041) (5.4189, 1.0021) (5.4268, 1.0001) (5.4347, 0.9981) (5.4427, 0.996) (5.4506, 0.9939) (5.4587, 0.9918) (5.4667, 0.9896) (5.4748, 0.9874) (5.483, 0.9851) (5.4911, 0.9828) (5.4993, 0.9804) (5.5076, 0.978) (5.5159, 0.9756) (5.5242, 0.9731) (5.5325, 0.9706) (5.5409, 0.968) (5.5493, 0.9654) (5.5577, 0.9628) (5.5662, 0.9601) (5.5747, 0.9574) (5.5833, 0.9546) (5.5919, 0.9518) (5.6005, 0.9489) (5.6091, 0.946) (5.6178, 0.9431) (5.6265, 0.9401) (5.6352, 0.9371) (5.644, 0.934) (5.6528, 0.9309) (5.6616, 0.9277) (5.6704, 0.9245) (5.6793, 0.9213) (5.6882, 0.918) (5.6971, 0.9146) (5.7061, 0.9113) (5.7151, 0.9078) (5.7241, 0.9044) (5.7331, 0.9008) (5.7422, 0.8973) (5.7513, 0.8937) (5.7604, 0.89) (5.7695, 0.8863) (5.7787, 0.8826) (5.7879, 0.8788) (5.7971, 0.875) (5.8063, 0.8711) (5.8156, 0.8672) (5.8249, 0.8632) (5.8342, 0.8592) (5.8435, 0.8551) (5.8529, 0.851) (5.8622, 0.8469) (5.8716, 0.8427) (5.881, 0.8384) (5.8905, 0.8341) (5.8999, 0.8298) (5.9094, 0.8254) (5.9189, 0.821) (5.9284, 0.8165) (5.938, 0.812) (5.9475, 0.8074) (5.9571, 0.8028) (5.9667, 0.7981) (5.9763, 0.7934) (5.9859, 0.7887) (5.9956, 0.7839) (6.0052, 0.779) (6.0149, 0.7741) (6.0246, 0.7692) (6.0343, 0.7642) (6.044, 0.7591) (6.0538, 0.754) (6.0635, 0.7489) (6.0733, 0.7437) (6.0831, 0.7385) (6.0929, 0.7332) (6.1027, 0.7279) (6.1126, 0.7225) (6.1224, 0.7171) (6.1323, 0.7116) (6.1421, 0.7061) (6.152, 0.7005) (6.1619, 0.6949) (6.1718, 0.6893) (6.1818, 0.6836) (6.1917, 0.6778) (6.2016, 0.672) (6.2116, 0.6661) (6.2216, 0.6602) (6.2316, 0.6543) (6.2415, 0.6483) (6.2515, 0.6423) (6.2616, 0.6362) (6.2716, 0.63) (6.2816, 0.6238) (6.2916, 0.6176) (6.3017, 0.6113) (6.3117, 0.605) (6.3218, 0.5986) (6.3319, 0.5921) (6.342, 0.5857) (6.3521, 0.5791) (6.3621, 0.5726) (6.3722, 0.5659) (6.3824, 0.5593) (6.3925, 0.5525) (6.4026, 0.5458) (6.4127, 0.5389) (6.4229, 0.5321) (6.433, 0.5252) (6.4431, 0.5182) (6.4533, 0.5112) (6.4634, 0.5041) (6.4736, 0.497) (6.4838, 0.4898) (6.4939, 0.4826) (6.5041, 0.4754) (6.5143, 0.4681) (6.5244, 0.4607) (6.5346, 0.4533) (6.5448, 0.4459) (6.555, 0.4384) (6.5652, 0.4308) (6.5754, 0.4232) (6.5855, 0.4156) (6.5957, 0.4079) (6.6059, 0.4001) (6.6161, 0.3923) (6.6263, 0.3845) (6.6365, 0.3766) (6.6447, 0.3702) (6.6508, 0.3655) (6.6549, 0.3623) (6.6569, 0.3607) knots 0 0 0 0 0 0 0.00416667 0.00833333 0.0125 0.01666667 0.02083333 0.025 0.02916667 0.03333333 0.0375 0.04166667 0.04583333 0.05 0.05416667 0.05833333 0.0625 0.06666667 0.07083333 0.075 0.07916667 0.08333333 0.0875 0.09166667 0.09583333 0.1 0.10416667 0.10833333 0.1125 0.11666667 0.12083333 0.125 0.12916667 0.13333333 0.1375 0.14166667 0.14583333 0.15 0.15416667 0.15833333 0.1625 0.16666667 0.17083333 0.175 0.17916667 0.18333333 0.1875 0.19166667 0.19583333 0.2 0.20416667 0.20833333 0.2125 0.21666667 0.22083333 0.225 0.22916667 0.23333333 0.2375 0.24166667 0.24583333 0.25 0.25416667 0.25833333 0.2625 0.26666667 0.27083333 0.275 0.27916667 0.28333333 0.2875 0.29166667 0.29583333 0.3 0.30416667 0.30833333 0.3125 0.31666667 0.32083333 0.325 0.32916667 0.33333333 0.3375 0.34166667 0.34583333 0.35 0.35416667 0.35833333 0.3625 0.36666667 0.37083333 0.375 0.37916667 0.38333333 0.3875 0.39166667 0.39583333 0.4 0.40416667 0.40833333 0.4125 0.41666667 0.42083333 0.425 0.42916667 0.43333333 0.4375 0.44166667 0.44583333 0.45 0.45416667 0.45833333 0.4625 0.46666667 0.47083333 0.475 0.47916667 0.48333333 0.4875 0.49166667 0.49583333 0.5 0.50416667 0.50833333 0.5125 0.51666667 0.52083333 0.525 0.52916667 0.53333333 0.5375 0.54166667 0.54583333 0.55 0.55416667 0.55833333 0.5625 0.56666667 0.57083333 0.575 0.57916667 0.58333333 0.5875 0.59166667 0.59583333 0.6 0.60416667 0.60833333 0.6125 0.61666667 0.62083333 0.625 0.62916667 0.63333333 0.6375 0.64166667 0.64583333 0.65 0.65416667 0.65833333 0.6625 0.66666667 0.67083333 0.675 0.67916667 0.68333333 0.6875 0.69166667 0.69583333 0.7 0.70416667 0.70833333 0.7125 0.71666667 0.72083333 0.725 0.72916667 0.73333333 0.7375 0.74166667 0.74583333 0.75 0.75416667 0.75833333 0.7625 0.76666667 0.77083333 0.775 0.77916667 0.78333333 0.7875 0.79166667 0.79583333 0.8 0.80416667 0.80833333 0.8125 0.81666667 0.82083333 0.825 0.82916667 0.83333333 0.8375 0.84166667 0.84583333 0.85 0.85416667 0.85833333 0.8625 0.86666667 0.87083333 0.875 0.87916667 0.88333333 0.8875 0.89166667 0.89583333 0.9 0.90416667 0.90833333 0.9125 0.91666667 0.92083333 0.925 0.92916667 0.93333333 0.9375 0.94166667 0.94583333 0.95 0.95416667 0.95833333 0.9625 0.96666667 0.97083333 0.975 0.97916667 0.98333333 0.9875 0.99166667 0.99583333 1 1 1 1 1 1
  spline S2 degree 5 poles (4.9003, -1.0509) (4.9003, -1.0509) (4.9004, -1.0509) (4.9005, -1.0509) (4.9006, -1.0509) (4.9008, -1.051) (4.9009, -1.051) (4.901, -1.051) (4.901, -1.051) (4.9011, -1.051) knots 0 0 0 0 0 0 0.2 0.4 0.6 0.8 1 1 1 1 1 1
  spline S3 degree 5 poles (4.9003, 1.0509) (4.9003, 1.0509) (4.9004, 1.0509) (4.9005, 1.0509) (4.9006, 1.0509) (4.9008, 1.051) (4.9009, 1.051) (4.901, 1.051) (4.901, 1.051) (4.9011, 1.051) knots 0 0 0 0 0 0 0.2 0.4 0.6 0.8 1 1 1 1 1 1
  line L0 (0, 0) -> (4.9003, -1.0509)
  line L1 (0, 0) -> (4.9003, 1.0509)
  arc A0 (6.6569, -0.3607) -> (6.6569, 0.3607) centre (0, 0) ccw
  point P0 (4.9034, -1.0515)
  point P1 (4.9074, -1.0521)
  point P2 (4.913, -1.053)
  point P3 (4.9201, -1.0539)
  point P4 (4.9289, -1.0549)
  point P5 (4.9393, -1.0559)
  point P6 (4.9513, -1.0568)
  point P7 (4.9649, -1.0576)
  point P8 (4.9802, -1.0582)
  point P9 (4.997, -1.0586)
  point P10 (5.0155, -1.0587)
  point P11 (5.0356, -1.0585)
  point P12 (5.0573, -1.0578)
  point P13 (5.0805, -1.0567)
  point P14 (5.1054, -1.055)
  point P15 (5.1318, -1.0528)
  point P16 (5.1597, -1.0499)
  point P17 (5.1892, -1.0464)
  point P18 (5.2203, -1.0421)
  point P19 (5.2528, -1.037)
  point P20 (5.2868, -1.031)
  point P21 (5.3223, -1.0241)
  point P22 (5.3592, -1.0163)
  point P23 (5.3975, -1.0074)
  point P24 (5.4373, -0.9975)
  point P25 (5.4784, -0.9864)
  point P26 (5.5208, -0.9741)
  point P27 (5.5645, -0.9606)
  point P28 (5.6096, -0.9459)
  point P29 (5.6558, -0.9298)
  point P30 (5.7033, -0.9123)
  point P31 (5.752, -0.8934)
  point P32 (5.8018, -0.873)
  point P33 (5.8527, -0.8511)
  point P34 (5.9046, -0.8276)
  point P35 (5.9576, -0.8025)
  point P36 (6.0116, -0.7758)
  point P37 (6.0665, -0.7474)
  point P38 (6.1223, -0.7172)
  point P39 (6.1789, -0.6852)
  point P40 (6.2364, -0.6514)
  point P41 (6.2946, -0.6157)
  point P42 (6.3535, -0.5782)
  point P43 (6.4131, -0.5387)
  point P44 (6.4733, -0.4972)
  point P45 (6.534, -0.4537)
  point P46 (6.5952, -0.4082)
  point P47 (4.9034, 1.0515)
  point P48 (4.9074, 1.0521)
  point P49 (4.913, 1.053)
  point P50 (4.9201, 1.0539)
  point P51 (4.9289, 1.0549)
  point P52 (4.9393, 1.0559)
  point P53 (4.9513, 1.0568)
  point P54 (4.9649, 1.0576)
  point P55 (4.9802, 1.0582)
  point P56 (4.997, 1.0586)
  point P57 (5.0155, 1.0587)
  point P58 (5.0356, 1.0585)
  point P59 (5.0573, 1.0578)
  point P60 (5.0805, 1.0567)
  point P61 (5.1054, 1.055)
  point P62 (5.1318, 1.0528)
  point P63 (5.1597, 1.0499)
  point P64 (5.1892, 1.0464)
  point P65 (5.2203, 1.0421)
  point P66 (5.2528, 1.037)
  point P67 (5.2868, 1.031)
  point P68 (5.3223, 1.0241)
  point P69 (5.3592, 1.0163)
  point P70 (5.3975, 1.0074)
  point P71 (5.4373, 0.9975)
  point P72 (5.4784, 0.9864)
  point P73 (5.5208, 0.9741)
  point P74 (5.5645, 0.9606)
  point P75 (5.6096, 0.9459)
  point P76 (5.6558, 0.9298)
  point P77 (5.7033, 0.9123)
  point P78 (5.752, 0.8934)
  point P79 (5.8018, 0.873)
  point P80 (5.8527, 0.8511)
  point P81 (5.9046, 0.8276)
  point P82 (5.9576, 0.8025)
  point P83 (6.0116, 0.7758)
  point P84 (6.0665, 0.7474)
  point P85 (6.1223, 0.7172)
  point P86 (6.1789, 0.6852)
  point P87 (6.2364, 0.6514)
  point P88 (6.2946, 0.6157)
  point P89 (6.3535, 0.5782)
  point P90 (6.4131, 0.5387)
  point P91 (6.4733, 0.4972)
  point P92 (6.534, 0.4537)
  point P93 (6.5952, 0.4082)
sketch "Sketch2" plane through (0, 0, 0) normal (0, 0, 1) x (1, 0, 0) in component "Component"
  circle A0 centre (0, 0) radius 3.6667
extrude "Extrude1" add sketch "Sketch2" along normal blind 3 makes body 1 in component "Component"
extrude "Extrude2" add sketch "Sketch1" along normal blind 3 separate body makes body 2 in component "Component"
pattern_circular "C-Pattern1" count 8 over 360 about axis through (0, 0, 1.75) along (0, 0, 1) of "Extrude2" makes body 3 at (1.4029, 0.9075, 1) makes body 4 at (0.7007, 3.2674, 2) makes body 5 at (-0.9075, 1.4029, 1) makes body 6 at (-1.6337, 0.3503, 1) makes body 7 at (-1.4029, -0.9075, 1) makes body 8 at (-0.3503, -1.6337, 1) makes body 9 at (0.9075, -1.4029, 1) in component "Component"
combine "Combine1" operation add target body 1 tool bodies 2 3 4 5 6 7 8 9 in component "Component"
sketch "Sketch3" plane through (0, 0, 0) normal (0, 0, 1) x (1, 0, 0) in component "Component"
  line L0 (0, 0) -> (50.8154, 0) construction
  line L1 (50.8154, 0) -> (50.8154, 3) construction
  line L2 (50.8154, 3) -> (0, 3) construction
  line L3 (0, 3) -> (0, 0) construction
  constraint perpendicular L0 L1
  constraint parallel L0 L2
  constraint parallel L1 L3